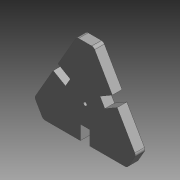
# Autodesk Inventor part: Lower Platform
Saved by Autodesk Inventor 2014 SP1 (Build 180222100, 222)
## iProperties
Created: 2013-12-29
Part Number: Lower Platform
Material: Generic
Document SubType Name: Modeling
Designer: tom
Density: 1 g/cm^3
Appearance: Default
Author: tom
Autodesk Inventor part; units mm, degrees
ref_plane "YZ Plane" through (0, 0, 0) normal (1, 0, 0) x (0, 1, 0)
ref_plane "XZ Plane" through (0, 0, 0) normal (0, 1, 0) x (-1, 0, 0)
ref_plane "XY Plane" through (0, 0, 0) normal (0, 0, 1) x (1, 0, 0)
sketch "Sketch1" plane through (0, 0, 0) normal (0, 0, 1) x (1, 0, 0)
  line L0 (0, 40) -> (34.641, -20)
  line L1 (34.641, -20) -> (-34.641, -20)
  line L2 (-34.641, -20) -> (0, 40)
  circle A0 centre (0, 0) radius 1
  dimension "d0" = 2
  dimension "d1" = 20
  constraints: 6 end point, 2 coincident, 1 centre point, 7 other
  measures "d0" diameter of A0
  measures "d1" distance from line of point (0, 0) L0
extrude "Extrusion1" add sketch "Sketch1" along normal blind 5.66
sketch "Sketch2" plane through (0, 0, 5.66) normal (0, 0, 1) x (1, 0, 0)
  circle A0 centre (0, 0) radius 1 projected
  line L0 (-34.641, -20) -> (34.641, -20) projected
  line L1 (0, -1) -> (0, 0)
  line L2 (-2.83, -11.66) -> (-2.83, -20)
  line L3 (2.83, -11.66) -> (2.83, -20)
  line L4 (2.83, -11.66) -> (-2.83, -11.66)
  point P0 (0, -20)
  dimension "d15" = 8.34
  dimension "d16" = 2.83
  dimension "d17" = 2.83
  constraints: 8 end point, 4 perpendicular, 2 point on line, 1 midpoint, 1 vertical alignment, 1 other
  measures "d15" distance between parallel lines of L0 L4
  measures "d16" distance from line of L3 L1.end
  measures "d17" distance from line of L1.end L2
extrude "Extrusion2" cut sketch "Sketch2" against normal blind 8.625
pattern_circular "Circular Pattern1" count 3 over 360 about axis through (0, 0, 0) along (0, 0, 1) of "Extrusion2"
chamfer "Chamfer1" distance 10 angle 45 3 edges at (34.641, -20, 2.83) (-34.641, -20, 2.83) (0, 40, 2.83)
fillet "Fillet1" radius 2 6 edges at (-29.641, -11.3397, 2.83) (-24.641, -20, 2.83) (-5, 31.3397, 2.83) (5, 31.3397, 2.83) (29.641, -11.3397, 2.83) (24.641, -20, 2.83)
body "Solid1"
